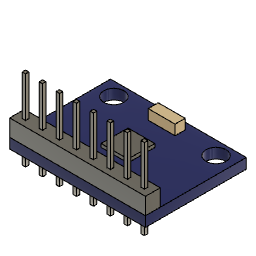
MPU6050 v3 (Autodesk Fusion 360 design; units mm, degrees)
Autodesk Fusion 360 part; units mm, degrees
sketch "base" plane through (0, 0, 0) normal (0, 0, 1) x (1, 0, 0)
  line L0 (-10.1, 7.5) -> (10.1, 7.5)
  line L1 (10.1, 7.5) -> (10.1, -7.5)
  line L2 (10.1, -7.5) -> (-10.1, -7.5)
  line L3 (-10.1, -7.5) -> (-10.1, 7.5)
  line L4 (0, 0) -> (30, 0) construction
  line L5 (0, 0) -> (0, 39.4345) construction
  circle A0 centre (-7.6, 5.5) radius 1.5
  circle A1 centre (7.6, 5.5) radius 1.5
  line L6 (-13.6828, -5.3) -> (15.1887, -5.3) construction
  line L7 (-10.1, -5.3) -> (-7.575, -5.3)
  line L8 (-7.575, -5.3) -> (-7.575, -7.5)
  line L9 (-7.575, -7.5) -> (-10.1, -7.5)
  line L10 (-10.1, -7.5) -> (-10.1, -5.3)
  line L11 (-5.05, -7.5) -> (-5.05, -18.9706) construction
  line L12 (-7.575, -5.3) -> (-5.05, -5.3) construction
  line L13 (-5.05, -5.3) -> (-5.05, -7.5) construction
  line L14 (-5.05, -7.5) -> (-7.575, -7.5) construction
  line L15 (-7.575, -7.5) -> (-7.575, -5.3) construction
  line L16 (-7.575, -5.3) -> (-5.05, -5.3)
  line L17 (-5.05, -5.3) -> (-5.05, -7.5)
  line L18 (-5.05, -7.5) -> (-7.575, -7.5)
  line L19 (-7.575, -7.5) -> (-7.575, -5.3)
  line L20 (-2.525, -7.5) -> (-2.525, -5.3)
  line L21 (-5.05, -5.3) -> (-2.525, -5.3)
  line L22 (-2.525, -5.3) -> (-2.525, -7.5)
  line L23 (-2.525, -7.5) -> (-5.05, -7.5)
  line L24 (-5.05, -7.5) -> (-5.05, -5.3)
  line L25 (-2.525, -5.3) -> (0, -5.3)
  line L26 (0, -5.3) -> (0, -7.5)
  line L27 (0, -7.5) -> (-2.525, -7.5)
  line L28 (-2.525, -7.5) -> (-2.525, -5.3)
  line L29 (-10.1, -5.3) -> (-7.575, -5.3)
  line L30 (-7.575, -5.3) -> (-7.575, -7.5)
  line L31 (-7.575, -7.5) -> (-10.1, -7.5)
  line L32 (-10.1, -7.5) -> (-10.1, -5.3)
  line L33 (10.1, -7.5) -> (10.1, -5.3)
  line L34 (7.575, -7.5) -> (10.1, -7.5)
  line L35 (10.1, -5.3) -> (7.575, -5.3)
  line L36 (7.575, -5.3) -> (7.575, -7.5)
  line L37 (7.575, -5.3) -> (5.05, -5.3)
  line L38 (5.05, -5.3) -> (5.05, -7.5)
  line L39 (2.525, -5.3) -> (2.525, -7.5)
  line L40 (5.05, -5.3) -> (2.525, -5.3)
  line L41 (13.6828, -5.3) -> (-15.1887, -5.3) construction
  line L42 (0, -5.3) -> (0, -7.5)
  line L43 (0, -7.5) -> (2.525, -7.5)
  line L44 (2.525, -7.5) -> (5.05, -7.5)
  line L45 (-10.1, -7.5) -> (10.1, -7.5)
  line L46 (0, -5.3) -> (2.525, -5.3)
  line L47 (2.525, -5.3) -> (2.525, -7.5)
  line L48 (2.525, -7.5) -> (0, -7.5)
  line L49 (0, -7.5) -> (0, -5.3)
  line L50 (-10.1, -6.4) -> (-7.575, -6.4) construction
  line L51 (-8.8375, -5.3) -> (-8.8375, -7.5) construction
  line L52 (-8.5875, -6.15) -> (-9.0875, -6.15)
  line L53 (-9.0875, -6.15) -> (-9.0875, -6.65)
  line L54 (-9.0875, -6.65) -> (-8.5875, -6.65)
  line L55 (-8.5875, -6.65) -> (-8.5875, -6.15)
  line L56 (-8.5875, -6.15) -> (-9.0875, -6.65) construction
  line L57 (-9.0875, -6.15) -> (-8.5875, -6.65) construction
  line L58 (-5.05, -6.4) -> (-7.575, -6.4) construction
  line L59 (-6.0625, -6.65) -> (-6.5625, -6.65)
  line L60 (-6.5625, -6.65) -> (-6.5625, -6.15)
  line L61 (-6.0625, -6.15) -> (-6.5625, -6.65) construction
  line L62 (-6.5625, -6.15) -> (-6.0625, -6.15)
  line L63 (-6.3125, -5.3) -> (-6.3125, -7.5) construction
  line L64 (-6.0625, -6.15) -> (-6.0625, -6.65)
  line L65 (-6.5625, -6.15) -> (-6.0625, -6.65) construction
  line L66 (-1.0125, -6.15) -> (-1.5125, -6.65) construction
  line L67 (-1.5125, -6.15) -> (-1.0125, -6.65) construction
  line L68 (-1.0125, -6.65) -> (-1.5125, -6.65)
  line L69 (-1.0125, -6.15) -> (-1.0125, -6.65)
  line L70 (-3.5375, -6.65) -> (-3.5375, -6.15)
  line L71 (-4.0375, -6.65) -> (-3.5375, -6.65)
  line L72 (-1.5125, -6.15) -> (-1.0125, -6.15)
  line L73 (-3.5375, -6.15) -> (-4.0375, -6.65) construction
  line L74 (-4.0375, -6.15) -> (-4.0375, -6.65)
  line L75 (-1.5125, -6.65) -> (-1.5125, -6.15)
  line L76 (-3.5375, -6.15) -> (-4.0375, -6.15)
  line L77 (-4.0375, -6.15) -> (-3.5375, -6.65) construction
  line L78 (3.5375, -6.15) -> (4.0375, -6.15)
  line L79 (6.0625, -6.15) -> (6.0625, -6.65)
  line L80 (6.5625, -6.15) -> (6.0625, -6.15)
  line L81 (3.5375, -6.65) -> (3.5375, -6.15)
  line L82 (6.5625, -6.65) -> (6.5625, -6.15)
  line L83 (4.0375, -6.15) -> (4.0375, -6.65)
  line L84 (6.0625, -6.65) -> (6.5625, -6.65)
  line L85 (4.0375, -6.15) -> (3.5375, -6.65) construction
  line L86 (3.5375, -6.15) -> (4.0375, -6.65) construction
  line L87 (4.0375, -6.65) -> (3.5375, -6.65)
  line L88 (6.5625, -6.15) -> (6.0625, -6.65) construction
  line L89 (6.0625, -6.15) -> (6.5625, -6.65) construction
  line L90 (9.0875, -6.15) -> (8.5875, -6.65) construction
  line L91 (8.5875, -6.15) -> (9.0875, -6.15)
  line L92 (8.5875, -6.15) -> (9.0875, -6.65) construction
  line L93 (8.5875, -6.65) -> (8.5875, -6.15)
  line L94 (9.0875, -6.15) -> (9.0875, -6.65)
  line L95 (9.0875, -6.65) -> (8.5875, -6.65)
  line L96 (5.05, -6.4) -> (7.575, -6.4) construction
  line L97 (1.0125, -6.65) -> (1.5125, -6.65)
  line L98 (1.5125, -6.65) -> (1.5125, -6.15)
  line L99 (1.5125, -6.15) -> (1.0125, -6.15)
  line L100 (1.0125, -6.15) -> (1.5125, -6.65) construction
  line L101 (1.0125, -6.15) -> (1.0125, -6.65)
  line L102 (1.5125, -6.15) -> (1.0125, -6.65) construction
  line L103 (-2, 6.5) -> (2, 6.5)
  line L104 (2, 6.5) -> (2, 5)
  line L105 (2, 5) -> (-2, 5)
  line L106 (-2, 5) -> (-2, 6.5)
  line L107 (-2, 6.5) -> (2, 5) construction
  line L108 (2, 6.5) -> (-2, 5) construction
  line L109 (-2, 2) -> (2, 2)
  line L110 (2, 2) -> (2, -2)
  line L111 (2, -2) -> (-2, -2)
  line L112 (-2, -2) -> (-2, 2)
  line L113 (-2, 2) -> (2, -2) construction
  line L114 (2, 2) -> (-2, -2) construction
  point P0 (-8.8375, -6.4)
  point P1 (-6.3125, -6.4)
  point P2 (-2.525, -6.4)
  point P3 (-2.525, -6.4)
  point P4 (-1.2625, -6.4)
  point P5 (-3.7875, -6.4)
  point P6 (7.575, -6.4)
  point P7 (1.2625, -6.4)
  point P8 (2.525, -6.4)
  point P9 (6.3125, -6.4)
  point P10 (8.8375, -6.4)
  point P11 (3.7875, -6.4)
  point P12 (2.525, -6.4)
  point P13 (0, 5.75)
  dimension "d1" = 20.2
  dimension "d2" = 15
  dimension "d3" = 30
  dimension "d4" = 7.5
  dimension "d5" = 10.1
  dimension "d6" = 3
  dimension "d7" = 2
  dimension "d8" = 2.5
  dimension "d9" = 2.2
  dimension "d10" = 2.525
  dimension "d11" = 5.05
  dimension "d12" = 0.5
  dimension "d13" = 0.5
  dimension "d14" = 4
  dimension "d15" = 1.5
  dimension "d16" = 1
  dimension "d27" = 4
  dimension "d28" = 4
  constraint horizontal L0
  constraint vertical L1
  constraint horizontal L2
  constraint vertical L3
  constraint coincident L4.start L5.start
  constraint perpendicular L1 L4
  constraint perpendicular L0 L5
  constraint symmetric L5 A0 A1
  constraint perpendicular L3 L6
  constraint horizontal L7
  constraint vertical L8
  constraint horizontal L9
  constraint vertical L10
  constraint coincident L3 L7.start
  constraint coincident L6 L7.start
  constraint coincident L2 L11.start
  constraint perpendicular L2 L11
  constraint horizontal L12
  constraint vertical L13
  constraint horizontal L14
  constraint vertical L15
  constraint horizontal L16
  constraint vertical L17
  constraint horizontal L18
  constraint vertical L19
  constraint symmetric L7.end L11 L20.end
  constraint symmetric L11 L8.end L20.start
  constraint horizontal L21
  constraint vertical L22
  constraint horizontal L23
  constraint vertical L24
  constraint horizontal L25
  constraint vertical L26
  constraint horizontal L27
  constraint vertical L28
  constraint midpoint L2 L26.end
  constraint horizontal L29
  constraint vertical L30
  constraint horizontal L31
  constraint vertical L32
  constraint symmetric L1.end L5 L2.end
  constraint symmetric L2.end L5 L1.end
  constraint symmetric L5 L6.start L41.start
  constraint symmetric L5 L6.end L41.end
  constraint symmetric L5 L7.start L33.end
  constraint symmetric L5 L7.end L35.end
  constraint symmetric L5 L8.end L34.start
  constraint symmetric L5 L2.end L1.end
  constraint symmetric L5 L11.start L38.end
  constraint symmetric L5 L12.end L37.end
  constraint symmetric L5 L20.start L39.end
  constraint symmetric L5 L20.end L39.start
  constraint symmetric L5 L25.end L26.start
  constraint symmetric L5 L26.end L27.start
  constraint horizontal L46
  constraint vertical L47
  constraint horizontal L48
  constraint vertical L49
  constraint midpoint L32 L50.start
  constraint midpoint L8 L50.end
  constraint midpoint L7 L51.start
  constraint midpoint L9 L51.end
  constraint perpendicular L52 L53
  constraint parallel L52 L54
  constraint parallel L53 L55
  constraint horizontal L52
  constraint coincident L56 P0
  constraint coincident L57 P0
  constraint midpoint L50 P0
  constraint symmetric L15 L50.start L58.start
  constraint symmetric L15 L50.end L58.end
  constraint symmetric L15 L51.start L63.start
  constraint symmetric L15 L51.end L63.end
  constraint symmetric L15 L52.start L60.end
  constraint symmetric L15 L52.end L61.start
  constraint symmetric L15 L53.end L59.start
  constraint symmetric L15 L54.end L59.end
  constraint symmetric L15 P0 P1
  constraint symmetric L24 L50.end P3
  constraint symmetric L24 L52.start L67.start
  constraint symmetric L24 L52.end L66.start
  constraint symmetric L24 L53.end L67.end
  constraint symmetric L24 L54.end L66.end
  constraint symmetric L24 P0 P4
  constraint symmetric L24 L60.end L70.end
  constraint symmetric L24 L61.start L74.start
  constraint symmetric L24 L59.start L71.start
  constraint symmetric L24 L59.end L70.start
  constraint symmetric L24 P1 P5
  constraint symmetric L42 L50.end P6
  constraint symmetric L42 L52.start L91.start
  constraint symmetric L42 L52.end L90.start
  constraint symmetric L42 L53.end L92.end
  constraint symmetric L42 L54.end L90.end
  constraint symmetric L42 P0 P10
  constraint symmetric L42 L60.end L80.start
  constraint symmetric L42 L61.start L79.start
  constraint symmetric L42 L59.start L79.end
  constraint symmetric L42 L59.end L82.start
  constraint symmetric L42 P1 P9
  constraint symmetric L42 L58.start L96.start
  constraint symmetric L42 L71.start L83.end
  constraint symmetric L42 L74.start L78.end
  constraint symmetric L42 L66.start L99.end
  constraint symmetric L42 L70.start L81.start
  constraint symmetric L42 L67.start L98.end
  constraint symmetric L42 P3 P12
  constraint symmetric L42 P4 P7
  constraint symmetric L42 L66.end L97.end
  constraint symmetric L42 L67.end L97.start
  constraint symmetric L42 L70.end L78.start
  constraint symmetric L42 P5 P11
  constraint perpendicular L103 L104
  constraint parallel L103 L105
  constraint parallel L104 L106
  constraint horizontal L103
  constraint coincident L107 P13
  constraint coincident L108 P13
  constraint coincident L5 P13
  constraint perpendicular L109 L110
  constraint parallel L109 L111
  constraint parallel L110 L112
  constraint horizontal L109
  constraint coincident L113 L4.start
  constraint coincident L114 L4.start
  measures "d1" distance of L0.start L0.end
  measures "d2" distance of L0.start L2.end
  measures "d3" distance of L4.start L4.end
  measures "d4" distance of L0 L4
  measures "d5" distance of L1 L5
  measures "d6" diameter of A0
  measures "d7" distance of L0 A0.centre
  measures "d8" distance of L3 A0.centre
  measures "d9" distance of L2 L6
  measures "d10" distance of L7.start L7.end
  measures "d11" distance of L5 L11
  measures "d12" distance of L53.end L54.end
  measures "d13" distance of L52.end L53.end
  measures "d14" distance of L104.end L105.end
  measures "d15" distance of L103.end L104.end
  measures "d16" distance of L0 L103
  measures "d27" distance of L110.end L111.end
  measures "d28" distance of L109.end L110.end
extrude "Extrude6" add sketch "base" along normal blind 0.5 contours L109 L110 L111 L112 makes body 1
extrude "Extrude4" add sketch "base" against normal blind 3.5 separate body contours L52 L53 L54 L55 | L59 L60 L62 L64 | L68 L69 L72 L75 | L70 L71 L74 L76 | L78 L81 L83 L87 | L79 L80 L82 L84 | L91 L93 L94 L95 | L97 L98 L99 L101 makes body 2 at (3.7042, -6.15, -1.1667) makes body 3 at (-6.2292, -6.65, -1.1667) makes body 4 at (-3.8708, -6.65, -1.1667) makes body 5 at (6.3958, -6.15, -1.1667) makes body 6 at (1.3458, -6.15, -1.1667) makes body 7 at (-8.5875, -6.4833, -1.1667) makes body 8 at (-1.1792, -6.65, -1.1667) makes body 9 at (8.7542, -6.15, -1.1667)
extrude "Extrude3" add sketch "base" along normal blind 8.5 separate body contours L52 L53 L54 L55 | L59 L60 L62 L64 | L68 L69 L72 L75 | L70 L71 L74 L76 | L78 L81 L83 L87 | L79 L80 L82 L84 | L91 L93 L94 L95 | L97 L98 L99 L101 makes body 10 at (3.7042, -6.15, 2.8333) makes body 11 at (-6.2292, -6.65, 2.8333) makes body 12 at (-3.8708, -6.65, 2.8333) makes body 13 at (6.3958, -6.15, 2.8333) makes body 14 at (1.3458, -6.15, 2.8333) makes body 15 at (-8.5875, -6.4833, 2.8333) makes body 16 at (-1.1792, -6.65, 2.8333) makes body 17 at (8.7542, -6.15, 2.8333)
extrude "Extrude2" add sketch "base" along normal blind 2.5 separate body contours L2 L3 L7 L8 L9 L10 L19 L29 L30 L31 L32 L45 | L1 L2 L33 L34 L35 L36 L45 | L2 L8 L16 L17 L18 L19 L24 L30 L45 | L2 L36 L37 L38 L45 | L2 L17 L20 L21 L22 L23 L24 L28 L45 | L2 L38 L39 L40 L44 L45 L47 | L2 L20 L22 L25 L26 L27 L28 L42 L45 L49 | L2 L26 L39 L42 L43 L45 L46 L47 L48 L49 makes body 18
extrude "Extrude1" add sketch "base" against normal blind 1.5 separate body contours L0 L1 L3 L7 L16 L21 L25 L29 L35 L37 L40 L46 | L2 L3 L7 L8 L9 L10 L19 L29 L30 L31 L32 L45 | L1 L2 L33 L34 L35 L36 L45 | L2 L8 L16 L17 L18 L19 L24 L30 L45 | L2 L36 L37 L38 L45 | L2 L17 L20 L21 L22 L23 L24 L28 L45 | L2 L38 L39 L40 L44 L45 L47 | L2 L20 L22 L25 L26 L27 L28 L42 L45 L49 | L2 L26 L39 L42 L43 L45 L46 L47 L48 L49 | L52 L53 L54 L55 | L59 L60 L62 L64 | L68 L69 L72 L75 | L70 L71 L74 L76 | L78 L81 L83 L87 | L79 L80 L82 L84 | L91 L93 L94 L95 | L97 L98 L99 L101 | L103 L104 L105 L106 | L109 L110 L111 L112 makes body 19
extrude "Extrude5" add sketch "base" along normal blind 1.5 separate body contours L103 L104 L105 L106 makes body 20
equation "d10 = ( 10.1 / 4 ) * 1 mm"
equation "d11 = ( 10.1 / 2 ) * 1 mm"
named bodies: "pcb", "pin_holder", "pin6", "pin2", "pin3", "pin7", "pin5", "pin1", "pin4", "pin8", "solder6", "solder2", "solder3", "solder7", "solder5", "solder1", "solder4", "solder8", "chip", "chip2"
